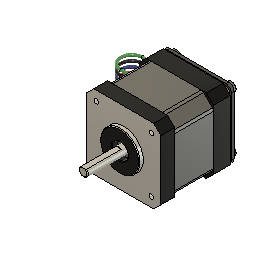
Nema 17 Closed loop v5 (Autodesk Fusion 360 design; units mm, degrees)
Autodesk Fusion 360 part; units mm, degrees
sketch "Sketch1" plane through (0, 0, 0) normal (0, 0, 1) x (1, 0, 0)
  line L0 (-20.9, 20.9) -> (20.9, 20.9)
  line L1 (20.9, 20.9) -> (20.9, -20.9)
  line L2 (20.9, -20.9) -> (-20.9, -20.9)
  line L3 (-20.9, -20.9) -> (-20.9, 20.9)
  line L4 (0, 20.9) -> (0, 0) construction
  line L5 (0, 0) -> (20.9, 0) construction
  dimension "d1" = 41.8
  dimension "d2" = 41.8
  constraint horizontal L0
  constraint vertical L1
  constraint horizontal L2
  constraint vertical L3
  constraint midpoint L0 L4.start
  constraint coincident L4.end L5.start
  constraint midpoint L1 L5.end
  constraint vertical L4
  constraint horizontal L5
  measures "d1" distance of L0.start L0.end
  measures "d2" distance of L0.end L1.end
extrude "Extrude1" add sketch "Sketch1" along normal blind 7.8 makes body 1
chamfer "Chamfer1" distance 4 angle 45 4 edges at (20.9, 20.9, 3.9) (-20.9, 20.9, 3.9) (20.9, -20.9, 3.9) (-20.9, -20.9, 3.9) on bodies 1
sketch "Sketch2" plane through (0, 0, 7.8) normal (0, 0, 1) x (1, 0, 0)
  line L0 (-20.9, -16.9) -> (-16.9, -20.9)
  line L1 (-16.9, -20.9) -> (16.9, -20.9)
  line L2 (16.9, -20.9) -> (20.9, -16.9)
  line L3 (20.9, -16.9) -> (20.9, 16.9)
  line L4 (20.9, 16.9) -> (16.9, 20.9)
  line L5 (16.9, 20.9) -> (-16.9, 20.9)
  line L6 (-16.9, 20.9) -> (-20.9, 16.9)
  line L7 (-20.9, 16.9) -> (-20.9, -16.9)
  circle A0 centre (0, 0) radius 11
  dimension "d6" = 22
  constraint coincident A0.centre origin
  measures "d6" diameter of A0
extrude "Extrude2" add sketch "Sketch2" along normal blind 2.3 contours A0 bodies 1
copy_body "Body->Comp1" bodies 1 removing the originals makes body 2 in component "Motor"
sketch "Sketch3" plane through (0, 0, 10.1) normal (0, 0, 1) x (1, 0, 0)
  circle A0 centre (0, 0) radius 4.5
  circle A1 centre (0, 0) radius 11
  dimension "d10" = 9
  constraint coincident A0.centre A1.centre
  measures "d10" diameter of A0
extrude "Extrude1'" cut sketch "Sketch3" against normal blind 3.5 contours A0 bodies 2 in component "Motor"
chamfer "Chamfer2" distance 0.4 angle 45 1 faces at (8.7924, -0.5465, 10.1) on bodies 2 in component "Motor"
sketch "Sketch4" plane through (0, 0, 6.6) normal (0, 0, 1) x (1, 0, 0)
  circle A0 centre (0, 0) radius 4.5
  circle A1 centre (0, 0) radius 2.5
  dimension "d14" = 5
  constraint coincident A0.centre A1.centre
  measures "d14" diameter of A1
extrude "Extrude3" add sketch "Sketch4" along normal blind 24 separate body contours A1 makes body 3
sketch "Sketch5" plane through (0, 0, 30.6) normal (0, 0, 1) x (1, 0, 0)
  circle A0 centre (0, 0) radius 2.5
  line L0 (-1.5, 2) -> (1.5, 2)
  line L1 (-7.396, -2.5) -> (6.5447, -2.5) construction
  dimension "d17" = 4.5
  constraint coincident A0 L0.start
  constraint coincident A0 L0.end
  constraint horizontal L0
  constraint parallel L0 L1
  constraint tangent A0 L1
  measures "d17" distance of L0 L1
extrude "Extrude4" cut sketch "Sketch5" against normal blind 20 contours A0 L0 picked at (-0.3999, 2.0645) bodies 3
chamfer "Chamfer2'" distance 0.4 angle 45 1 edges at (0, -2.5, 30.6) on bodies 3
sketch "Sketch6" plane through (0, 0, 7.8) normal (0, 0, 1) x (1, 0, 0)
  circle A0 centre (0, 0) radius 11
  line L0 (-20.9, -16.9) -> (-16.9, -20.9)
  line L1 (-16.9, -20.9) -> (16.9, -20.9)
  line L2 (16.9, -20.9) -> (20.9, -16.9)
  line L3 (20.9, -16.9) -> (20.9, 16.9)
  line L4 (20.9, 16.9) -> (16.9, 20.9)
  line L5 (16.9, 20.9) -> (-16.9, 20.9)
  line L6 (-16.9, 20.9) -> (-20.9, 16.9)
  line L7 (-20.9, 16.9) -> (-20.9, -16.9)
  circle A1 centre (-15.5, -15.5) radius 1.25
  circle A2 centre (15.5, -15.5) radius 1.25
  circle A3 centre (15.5, 15.5) radius 1.25
  circle A4 centre (-15.5, 15.5) radius 1.25
  dimension "d21" = 15.5
  dimension "d22" = 15.5
  dimension "d23" = 2.5
  dimension "d25" = 360
  measures "d21" horizontal distance of A0.centre A1.centre
  measures "d22" vertical distance of A0.centre A1.centre
  measures "d23" diameter of A1
extrude "Extrude2'" cut sketch "Sketch6" against normal blind 2.8 contours A1 | A2 | A3 | A4 bodies 2 in component "Motor"
copy_body "CutPasteBodies1" bodies 3 removing the originals makes body 4 in component "Motor"
sketch "Sketch1 (2)" plane through (0, 0, 0) normal (0, 0, -1) x (-1, 0, 0) in component "Motor"
  line L0 (16.9, -20.9) -> (20.9, -16.9)
  line L1 (20.9, -16.9) -> (20.9, 16.9)
  line L2 (20.9, 16.9) -> (16.9, 20.9)
  line L3 (16.9, 20.9) -> (-16.9, 20.9)
  line L4 (-16.9, 20.9) -> (-20.9, 16.9)
  line L5 (-20.9, 16.9) -> (-20.9, -16.9)
  line L6 (-20.9, -16.9) -> (-16.9, -20.9)
  line L7 (-16.9, -20.9) -> (16.9, -20.9)
  line L8 (-14.7787, 20.9) -> (-20.9, 14.7787)
  line L9 (-20.9, -14.7787) -> (-14.7787, -20.9)
  line L10 (14.7787, -20.9) -> (20.9, -14.7787)
  line L11 (20.9, 14.7787) -> (14.7787, 20.9)
  dimension "d28" = 1.5
  dimension "d30" = 360
  constraint coincident L3 L8.start
  constraint coincident L5 L8.end
  constraint parallel L4 L8
  measures "d28" distance of L4 L8
extrude "Extrude3'" add sketch "Sketch1 (2)" along normal blind 21.85 separate body contours L1 L3 L5 L7 L8 L9 L10 L11 makes body 5 in component "Motor"
fillet "Fillet1" radius 2 8 edges at (-14.7787, 20.9, -10.925) (-20.9, 14.7787, -10.925) (-20.9, -14.7787, -10.925) (-14.7787, -20.9, -10.925) (14.7787, 20.9, -10.925) (20.9, 14.7787, -10.925) (20.9, -14.7787, -10.925) (14.7787, -20.9, -10.925) on bodies 5 in component "Motor"
sketch "Sketch2 (2)" plane through (0, 0, -21.85) normal (0, 0, -1) x (-1, 0, 0) in component "Motor"
  arc A0 (-15.3645, -20.3142) -> (-13.9503, -20.9) centre (-13.9503, -18.9) ccw
  line L0 (-13.9503, -20.9) -> (13.9503, -20.9)
  arc A1 (13.9503, -20.9) -> (15.3645, -20.3142) centre (13.9503, -18.9) ccw
  line L1 (15.3645, -20.3142) -> (20.3142, -15.3645)
  arc A2 (20.3142, -15.3645) -> (20.9, -13.9503) centre (18.9, -13.9503) ccw
  line L2 (20.9, -13.9503) -> (20.9, 13.9503)
  arc A3 (20.9, 13.9503) -> (20.3142, 15.3645) centre (18.9, 13.9503) ccw
  line L3 (20.3142, 15.3645) -> (15.3645, 20.3142)
  arc A4 (15.3645, 20.3142) -> (13.9503, 20.9) centre (13.9503, 18.9) ccw
  line L4 (13.9503, 20.9) -> (-13.9503, 20.9)
  arc A5 (-13.9503, 20.9) -> (-15.3645, 20.3142) centre (-13.9503, 18.9) ccw
  line L5 (-15.3645, 20.3142) -> (-20.3142, 15.3645)
  arc A6 (-20.3142, 15.3645) -> (-20.9, 13.9503) centre (-18.9, 13.9503) ccw
  line L6 (-20.9, 13.9503) -> (-20.9, -13.9503)
  arc A7 (-20.9, -13.9503) -> (-20.3142, -15.3645) centre (-18.9, -13.9503) ccw
  line L7 (-20.3142, -15.3645) -> (-15.3645, -20.3142)
  line L8 (16.9, -20.9) -> (20.9, -16.9)
  line L9 (20.9, -16.9) -> (20.9, 16.9)
  line L10 (20.9, 16.9) -> (16.9, 20.9)
  line L11 (16.9, 20.9) -> (-16.9, 20.9)
  line L12 (-16.9, 20.9) -> (-20.9, 16.9)
  line L13 (-20.9, 16.9) -> (-20.9, -16.9)
  line L14 (-20.9, -16.9) -> (-16.9, -20.9)
  line L15 (-16.9, -20.9) -> (16.9, -20.9)
extrude "Extrude4'" add sketch "Sketch2 (2)" along normal blind 9.5 separate body makes body 6 in component "Motor"
sketch "Sketch3 (2)" plane through (-20.9, 0, 0) normal (-1, 0, 0) x (0, 0, 1) in component "Motor"
  line L0 (-21.85, -16.9) -> (-21.85, 16.9)
  line L1 (-21.85, 16.9) -> (-31.35, 16.9)
  line L2 (-31.35, 16.9) -> (-31.35, -16.9)
  line L3 (-31.35, -16.9) -> (-21.85, -16.9)
  line L4 (-31.35, 8.25) -> (-29.05, 8.25)
  line L5 (-29.05, 8.25) -> (-29.05, -8.25)
  line L6 (-29.05, -8.25) -> (-31.35, -8.25)
  line L7 (-31.35, -8.25) -> (-31.35, 8.25)
  line L8 (-29.05, 0) -> (0, 0) construction
  dimension "d37" = 16.5
  dimension "d38" = 2.3
  constraint horizontal L4
  constraint vertical L5
  constraint horizontal L6
  constraint vertical L7
  constraint coincident L2 L4.start
  constraint midpoint L5 L8.start
  constraint coincident L8.end origin
  constraint horizontal L8
  measures "d37" distance of L4.end L5.end
  measures "d38" distance of L4.start L4.end
extrude "Extrude5" add sketch "Sketch3 (2)" along normal blind 4 contours L2 L4 L5 L6 L7 bodies 6 in component "Motor"
sketch "Sketch4 (2)" plane through (-20.9, 0, 0) normal (-1, 0, 0) x (0, 0, 1) in component "Motor"
  line L0 (-31.35, 8.25) -> (-29.05, 8.25)
  line L1 (-29.05, 8.25) -> (-29.05, -8.25)
  line L2 (-29.05, -8.25) -> (-31.35, -8.25)
  line L3 (-31.35, -8.25) -> (-31.35, -16.9)
  line L4 (-31.35, -16.9) -> (-21.85, -16.9)
  line L5 (-21.85, -16.9) -> (-21.85, 16.9)
  line L6 (-21.85, 16.9) -> (-31.35, 16.9)
  line L7 (-31.35, 16.9) -> (-31.35, 8.25)
  line L8 (-29.05, 8.25) -> (-21.85, 8.25)
  line L9 (-21.85, 8.25) -> (-21.85, -8.25)
  line L10 (-21.85, -8.25) -> (-29.05, -8.25)
  line L11 (-29.05, -8.25) -> (-29.05, 8.25)
  constraint horizontal L8
  constraint vertical L9
  constraint horizontal L10
  constraint vertical L11
  constraint coincident L5 L9.end
  constraint coincident L0.end L1.start
  constraint collinear L2 L10
extrude "Extrude6" cut sketch "Sketch4 (2)" against normal blind 2 contours L1 L5 L8 L9 L10 L11 bodies 6 in component "Motor"
sketch "Sketch5 (2)" plane through (-18.9, 0, 0) normal (-1, 0, 0) x (0, 0, 1) in component "Motor"
  line L0 (-29.05, -8.25) -> (-21.85, -8.25)
  line L1 (-21.85, -8.25) -> (-21.85, 8.25)
  line L2 (-21.85, 8.25) -> (-29.05, 8.25)
  line L3 (-29.05, 8.25) -> (-29.05, -8.25)
  line L4 (-28.55, 7.75) -> (-22.35, 7.75)
  line L5 (-22.35, 7.75) -> (-22.35, -7.75)
  line L6 (-22.35, -7.75) -> (-28.55, -7.75)
  line L7 (-28.55, -7.75) -> (-28.55, 7.75)
  dimension "d43" = 0.5
  dimension "d44" = 0.5
  dimension "d45" = 0.5
  dimension "d46" = 0.5
  constraint horizontal L4
  constraint vertical L5
  constraint horizontal L6
  constraint vertical L7
  measures "d43" distance of L3 L7
  measures "d44" distance of L1 L5
  measures "d45" distance of L2 L4
  measures "d46" distance of L0 L6
extrude "Extrude7" add sketch "Sketch5 (2)" along normal blind 5 separate body contours L4 L5 L6 L7 makes body 7 in component "Motor"
sketch "Sketch6 (2)" plane through (0, 0, -31.35) normal (0, 0, -1) x (-1, 0, 0) in component "Motor"
  line L0 (-16.9, -20.9) -> (16.9, -20.9)
  line L1 (16.9, -20.9) -> (20.9, -16.9)
  line L2 (20.9, -16.9) -> (20.9, -8.25)
  line L3 (20.9, -8.25) -> (24.9, -8.25)
  line L4 (24.9, -8.25) -> (24.9, 8.25)
  line L5 (24.9, 8.25) -> (20.9, 8.25)
  line L6 (20.9, 8.25) -> (20.9, 16.9)
  line L7 (20.9, 16.9) -> (16.9, 20.9)
  line L8 (16.9, 20.9) -> (-16.9, 20.9)
  line L9 (-16.9, 20.9) -> (-20.9, 16.9)
  line L10 (-20.9, 16.9) -> (-20.9, -16.9)
  line L11 (-20.9, -16.9) -> (-16.9, -20.9)
  circle A0 centre (15.5, 15.5) radius 3.25
  circle A1 centre (15.5, 15.5) radius 1.25
  circle A2 centre (-15.5, 15.5) radius 3.25
  circle A3 centre (-15.5, -15.5) radius 3.25
  circle A4 centre (15.5, -15.5) radius 3.25
  dimension "d49" = 6.5
  dimension "d51" = 360
  constraint concentric A0 A1
  measures "d49" diameter of A0
extrude "Extrude8" add sketch "Sketch6 (2)" along normal blind 1.9 separate body contours A0 | A1 | A2 | A3 | A4 makes body 8 at (12.254, -15.662, -32.6167) makes body 9 at (12.254, 15.338, -32.6167) makes body 10 at (-18.746, -15.662, -32.6167) makes body 11 at (-18.746, 15.338, -32.6167) in component "Motor"
sketch "Sketch7" plane through (0, 0, -33.25) normal (0, 0, -1) x (-1, 0, 0) in component "Motor"
  circle A0 centre (15.5, 15.5) radius 3.25
  line L0 (-16.5, 19.5) -> (16.5, 19.5)
  line L1 (19.5, 16.5) -> (19.5, -16.5)
  line L2 (16.5, -19.5) -> (-16.5, -19.5)
  line L3 (-19.5, -16.5) -> (-19.5, 16.5)
  line L4 (16.9, 20.9) -> (-16.9, 20.9)
  line L5 (-16.9, -20.9) -> (16.9, -20.9)
  line L6 (-20.9, 16.9) -> (-20.9, -16.9)
  arc A1 (19.5, 16.5) -> (16.5, 19.5) centre (16.5, 16.5) ccw
  arc A2 (16.5, -19.5) -> (19.5, -16.5) centre (16.5, -16.5) ccw
  arc A3 (-19.5, -16.5) -> (-16.5, -19.5) centre (-16.5, -16.5) ccw
  arc A4 (-16.5, 19.5) -> (-19.5, 16.5) centre (-16.5, 16.5) ccw
  point P0 (-19.5, 19.5)
  point P1 (19.5, 19.5)
  point P2 (19.5, -19.5)
  dimension "d54" = 39
  dimension "d55" = 39
  dimension "d56" = 1.4
  dimension "d57" = 1.4
  dimension "d58" = 1.4
  dimension "d59" = 3
  constraint horizontal L0
  constraint vertical L1
  constraint horizontal L2
  constraint vertical L3
  constraint coincident P1 L0
  constraint coincident P1 L1
  constraint tangent L0 A1
  constraint tangent L1 A1
  constraint coincident P2 L1
  constraint coincident P2 L2
  constraint tangent L1 A2
  constraint tangent L2 A2
  constraint equal A1 A2
  constraint tangent L2 A3
  constraint tangent L3 A3
  constraint equal A1 A3
  constraint coincident P0 L0
  constraint coincident P0 L3
  constraint tangent L0 A4
  constraint tangent L3 A4
  constraint equal A1 A4
  measures "d54" distance of P0 P1
  measures "d55" distance of P1 P2
  measures "d56" distance of L0 L4
  measures "d57" distance of L2 L5
  measures "d58" distance of L3 L6
  measures "d59" radius of A1
extrude "Extrude9" add sketch "Sketch7" along normal blind 1.6 separate body contours A0 | L0 L1 L2 L3 A1 A2 A3 A4 makes body 12 in component "Motor"
sketch "Sketch8" plane through (0, 0, -34.85) normal (0, 0, -1) x (-1, 0, 0) in component "Motor"
  arc A0 (19.5, 16.5) -> (16.5, 19.5) centre (16.5, 16.5) ccw
  line L0 (16.5, 19.5) -> (-16.5, 19.5)
  arc A1 (-16.5, 19.5) -> (-19.5, 16.5) centre (-16.5, 16.5) ccw
  line L1 (-19.5, 16.5) -> (-19.5, -16.5)
  arc A2 (-19.5, -16.5) -> (-16.5, -19.5) centre (-16.5, -16.5) ccw
  line L2 (-16.5, -19.5) -> (16.5, -19.5)
  arc A3 (16.5, -19.5) -> (19.5, -16.5) centre (16.5, -16.5) ccw
  line L3 (19.5, -16.5) -> (19.5, 16.5)
  line L4 (18.4811, 6.25) -> (23.9, 6.25)
  line L5 (23.9, 6.25) -> (23.9, -6.25)
  line L6 (23.9, -6.25) -> (18.4811, -6.25)
  line L7 (18.4811, -6.25) -> (18.4811, 6.25)
  line L8 (23.9, 7.75) -> (23.9, -7.75)
  line L9 (0, 0) -> (18.4811, 0) construction
  dimension "d62" = 12.5
  dimension "d63" = 5.4189
  constraint horizontal L4
  constraint vertical L5
  constraint horizontal L6
  constraint vertical L7
  constraint collinear L5 L8
  constraint coincident L9.start origin
  constraint midpoint L7 L9.end
  constraint horizontal L9
  measures "d62" distance of L4.start L6.end
  measures "d63" distance of L4.start L4.end
extrude "Extrude10" add sketch "Sketch8" along normal blind 5.6 separate body contours L3 L4 L5 L6 L8 | L3 L4 L6 L7 makes body 13 in component "Motor"
ref_plane "WorkPlane1" through (-21.1906, -4.25, -37.65) normal (0, -1, 0) x (-1, 0, 0) in component "Motor"
sketch "Sketch9" plane through (-21.1906, -4.25, -37.65) normal (0, -1, 0) x (1, 0, 0) in component "Motor"
  line L0 (-2.7094, 0) -> (-13.6094, 0)
  line L1 (-2.7094, 12.2) -> (-13.6094, 12.2)
  line L2 (2.2906, 15.3) -> (-2.7094, 15.3)
  line L3 (2.7094, -2.8) -> (-2.7094, -2.8)
  line L4 (-2.7094, 9.1) -> (-2.7094, 15.3)
  line L5 (-2.7094, 2.8) -> (-2.7094, -2.8)
  arc A0 (-13.6094, 12.2) -> (-13.6094, 0) centre (-13.6094, 6.1) ccw
  line L6 (0.2906, 15.8) -> (0.2906, 6.3)
  point P0 (-19.7094, 6.1)
  dimension "d67" = 3.1
  dimension "d68" = 2.8
  dimension "d69" = 20
  constraint horizontal L0
  constraint parallel L0 L1
  constraint coincident L1.start L4
  constraint coincident L0.start L5
  constraint vertical L0.end L1.end
  constraint tangent L1 A0
  constraint midpoint A0 P0
  measures "d67" distance of L1 L2
  measures "d68" distance of L0 L3
  measures "d69" distance of P0 L6
sketch "Sketch10" plane through (-23.9, 0, 0) normal (-1, 0, 0) x (0, 0, 1) in component "Motor"
  line L0 (-34.85, -6.25) -> (-34.85, 6.25)
  line L1 (-34.85, 6.25) -> (-40.45, 6.25)
  line L2 (-40.45, 6.25) -> (-40.45, -6.25)
  line L3 (-40.45, -6.25) -> (-34.85, -6.25)
  circle A0 centre (-37.65, -4.25) radius 0.75
  point P0 (-37.65, -4.25)
  dimension "d70" = 1.5
  constraint coincident P0 A0.centre
  measures "d70" diameter of A0
sweep "Sweep1" add profiles "Sketch10" path "Sketch9" along L0 A0 L1 section 1 contours A0 separate body makes body 14 in component "Motor"
pattern_linear "R-Pattern1" count 4 spacing 2.9113 along (0, 1, 0) of bodies 14 makes body 15 at (-38.3482, -1.0822, -37.3564) makes body 16 at (-38.3482, 1.8292, -37.3564) makes body 17 at (-38.3482, 4.7405, -37.3564) in component "Motor"
sketch "Sketch11" plane through (0, 0, -34.85) normal (0, 0, -1) x (-1, 0, 0) in component "Motor"
  arc A0 (19.5, 16.5) -> (16.5, 19.5) centre (16.5, 16.5) ccw
  line L0 (16.5, 19.5) -> (-16.5, 19.5)
  arc A1 (-16.5, 19.5) -> (-19.5, 16.5) centre (-16.5, 16.5) ccw
  line L1 (-19.5, 16.5) -> (-19.5, -16.5)
  arc A2 (-19.5, -16.5) -> (-16.5, -19.5) centre (-16.5, -16.5) ccw
  line L2 (-16.5, -19.5) -> (16.5, -19.5)
  arc A3 (16.5, -19.5) -> (19.5, -16.5) centre (16.5, -16.5) ccw
  line L3 (19.5, -16.5) -> (19.5, 16.5)
  circle A4 centre (-15.5, 15.5) radius 2.725
  circle A5 centre (-15.5, -15.5) radius 2.725
  circle A6 centre (15.5, -15.5) radius 2.725
  circle A7 centre (15.5, 15.5) radius 2.725
  dimension "d81" = 5.45
  dimension "d82" = 4
  dimension "d83" = 4
  dimension "d85" = 360
  measures "d81" diameter of A4
  measures "d82" distance of L0 A4.centre
  measures "d83" distance of L1 A4.centre
extrude "Extrude11" add sketch "Sketch11" along normal blind 2.7 separate body contours A4 | A5 | A6 | A7 makes body 18 at (12.7784, 15.3642, -36.65) makes body 19 at (12.7784, -15.6358, -36.65) makes body 20 at (-18.2216, 15.3642, -36.65) makes body 21 at (-18.2216, -15.6358, -36.65) in component "Motor"
chamfer "Chamfer3" distance 0.3 angle 45 4 faces at (12.7784, -15.6358, -36.65) (12.7784, 15.3642, -36.65) (-18.2216, 15.3642, -36.65) (-18.2216, -15.6358, -36.65) on bodies 18 19 20 21 in component "Motor"
sketch "Sketch12" plane through (0, 0, -37.55) normal (0, 0, -1) x (-1, 0, 0) in component "Motor"
  circle A0 centre (-15.5, 15.5) radius 2.425
  line L0 (-14.25, 14.7783) -> (-14.25, 16.2217)
  line L1 (-14.25, 16.2217) -> (-15.5, 16.9434)
  line L2 (-15.5, 16.9434) -> (-16.75, 16.2217)
  line L3 (-16.75, 16.2217) -> (-16.75, 14.7783)
  line L4 (-16.75, 14.7783) -> (-15.5, 14.0566)
  line L5 (-15.5, 14.0566) -> (-14.25, 14.7783)
  line L6 (-16.9434, -15.5) -> (-16.2217, -16.75)
  line L7 (-16.2217, -14.25) -> (-16.9434, -15.5)
  line L8 (-14.7783, -14.25) -> (-16.2217, -14.25)
  line L9 (-14.0566, -15.5) -> (-14.7783, -14.25)
  line L10 (-14.7783, -16.75) -> (-14.0566, -15.5)
  line L11 (-16.2217, -16.75) -> (-14.7783, -16.75)
  line L12 (15.5, -16.9434) -> (16.75, -16.2217)
  line L13 (14.25, -16.2217) -> (15.5, -16.9434)
  line L14 (14.25, -14.7783) -> (14.25, -16.2217)
  line L15 (15.5, -14.0566) -> (14.25, -14.7783)
  line L16 (16.75, -14.7783) -> (15.5, -14.0566)
  line L17 (16.75, -16.2217) -> (16.75, -14.7783)
  line L18 (16.9434, 15.5) -> (16.2217, 16.75)
  line L19 (16.2217, 14.25) -> (16.9434, 15.5)
  line L20 (14.7783, 14.25) -> (16.2217, 14.25)
  line L21 (14.0566, 15.5) -> (14.7783, 14.25)
  line L22 (14.7783, 16.75) -> (14.0566, 15.5)
  line L23 (16.2217, 16.75) -> (14.7783, 16.75)
  point P0 (-15.5, 15.5)
  point P1 (-15.5, -15.5)
  point P2 (-15.5, -15.5)
  point P3 (15.5, -15.5)
  point P4 (15.5, -15.5)
  point P5 (15.5, 15.5)
  point P6 (15.5, 15.5)
  dimension "d89" = 2.5
  dimension "d91" = 360
  constraint coincident P0 A0.centre
  constraint vertical L0
  measures "d89" distance of L0 L3
extrude "Extrude12" cut sketch "Sketch12" against normal blind 2 contours L0 L1 L2 L3 L4 L5 | L6 L7 L8 L9 L10 L11 | L12 L13 L14 L15 L16 L17 | L18 L19 L20 L21 L22 L23 bodies 18 19 20 21 in component "Motor"
sketch "Sketch13" plane through (0, 0, -34.85) normal (0, 0, -1) x (-1, 0, 0) in component "Motor"
  arc A0 (19.5, 16.5) -> (16.5, 19.5) centre (16.5, 16.5) ccw
  line L0 (16.5, 19.5) -> (-16.5, 19.5)
  arc A1 (-16.5, 19.5) -> (-19.5, 16.5) centre (-16.5, 16.5) ccw
  line L1 (-19.5, 16.5) -> (-19.5, -16.5)
  arc A2 (-19.5, -16.5) -> (-16.5, -19.5) centre (-16.5, -16.5) ccw
  line L2 (-16.5, -19.5) -> (16.5, -19.5)
  arc A3 (16.5, -19.5) -> (19.5, -16.5) centre (16.5, -16.5) ccw
  line L3 (19.5, -16.5) -> (19.5, 16.5)
  line L4 (-8.75, -16.7) -> (8.75, -16.7)
  line L5 (8.75, -16.7) -> (8.75, -23.7)
  line L6 (8.75, -23.7) -> (-8.75, -23.7)
  line L7 (-8.75, -23.7) -> (-8.75, -16.7)
  line L8 (0, -16.7) -> (0, 0) construction
  line L9 (-16.9, -20.9) -> (16.9, -20.9)
  dimension "d94" = 17.5
  dimension "d95" = 7
  dimension "d96" = 2.8
  constraint horizontal L4
  constraint vertical L5
  constraint horizontal L6
  constraint vertical L7
  constraint midpoint L4 L8.start
  constraint coincident L8.end origin
  constraint vertical L8
  measures "d94" distance of L4.start L4.end
  measures "d95" distance of L4.end L5.end
  measures "d96" distance of L6 L9
extrude "Extrude13" add sketch "Sketch13" along normal blind 5.7 separate body contours L2 L5 L7 L9 | L2 L4 L5 L7 | L5 L6 L7 L9 makes body 22 in component "Motor"
sketch "Sketch14" plane through (0, -23.7, 0) normal (0, -1, 0) x (1, 0, 0) in component "Motor"
  line L0 (8.75, -34.85) -> (-8.75, -34.85)
  line L1 (-8.75, -34.85) -> (-8.75, -40.55)
  line L2 (-8.75, -40.55) -> (8.75, -40.55)
  line L3 (8.75, -40.55) -> (8.75, -34.85)
  line L4 (-8.05, -35.55) -> (8.05, -35.55)
  line L5 (8.05, -35.55) -> (8.05, -39.85)
  line L6 (-8.05, -39.85) -> (-8.05, -35.55)
  line L7 (-5, -39.85) -> (-5, -40.55)
  line L8 (-5, -40.55) -> (-6.5, -40.55)
  line L9 (-6.5, -40.55) -> (-6.5, -39.85)
  line L10 (6.5, -39.85) -> (6.5, -40.55)
  line L11 (6.5, -40.55) -> (5, -40.55)
  line L12 (5, -40.55) -> (5, -39.85)
  line L13 (-6.5, -39.85) -> (-8.05, -39.85)
  line L14 (8.05, -39.85) -> (6.5, -39.85)
  line L15 (5, -39.85) -> (-5, -39.85)
  dimension "d99" = 0.7
  dimension "d100" = 0.7
  dimension "d101" = 0.7
  dimension "d102" = 0.7
  dimension "d103" = 1.5
  dimension "d104" = 1.5
  dimension "d105" = 10
  constraint horizontal L4
  constraint vertical L5
  constraint horizontal L14
  constraint vertical L6
  constraint vertical L7
  constraint horizontal L8
  constraint vertical L9
  constraint coincident L2 L7.end
  constraint coincident L9.end L14
  constraint vertical L10
  constraint horizontal L11
  constraint vertical L12
  constraint coincident L2 L10.end
  constraint coincident L12.end L14
  constraint collinear L13 L14
  constraint collinear L14 L15
  constraint equal L13 L14
  measures "d99" distance of L1 L6
  measures "d100" distance of L3 L5
  measures "d101" distance of L2 L14
  measures "d102" distance of L0 L4
  measures "d103" distance of L10.end L11.end
  measures "d104" distance of L7.end L8.end
  measures "d105" distance of L7.start L12.end
extrude "Extrude14" cut sketch "Sketch14" against normal blind 5.5 contours L2 L4 L5 L6 L7 L8 L9 L10 L11 L12 L13 L14 L15 bodies 22 in component "Motor"
sketch "Sketch15" plane through (0, 0, -34.85) normal (0, 0, -1) x (-1, 0, 0) in component "Motor"
  arc A0 (19.5, 16.5) -> (16.5, 19.5) centre (16.5, 16.5) ccw
  line L0 (16.5, 19.5) -> (-16.5, 19.5)
  arc A1 (-16.5, 19.5) -> (-19.5, 16.5) centre (-16.5, 16.5) ccw
  line L1 (-19.5, 16.5) -> (-19.5, -16.5)
  arc A2 (-19.5, -16.5) -> (-16.5, -19.5) centre (-16.5, -16.5) ccw
  line L2 (-16.5, -19.5) -> (16.5, -19.5)
  arc A3 (16.5, -19.5) -> (19.5, -16.5) centre (16.5, -16.5) ccw
  line L3 (19.5, -16.5) -> (19.5, 16.5)
  line L4 (-2.5, 6) -> (5.5, 6)
  line L5 (5.5, 6) -> (5.5, -6)
  line L6 (5.5, -6) -> (-2.5, -6)
  line L7 (-2.5, -6) -> (-2.5, 6)
  dimension "d108" = 12
  dimension "d109" = 8
  dimension "d110" = 6
  dimension "d111" = 14
  constraint horizontal L4
  constraint vertical L5
  constraint horizontal L6
  constraint vertical L7
  measures "d108" distance of L4.start L6.end
  measures "d109" distance of L5.end L6.end
  measures "d110" distance of origin L6
  measures "d111" distance of L3 L5
extrude "Extrude15" add sketch "Sketch15" along normal blind 1.5 contours L4 L5 L6 L7 bodies 12 in component "Motor"
component "Motor" placed x (1, 0, 0) y (0, 1, 0) z (0, 0, 1) at (0, 0, 0)
equation "d25 = 360.0 °"
equation "d30 = 360.0 °"
equation "d51 = 360.0 °"
equation "d85 = 360.0 °"
equation "d91 = 360.0 °"
named bodies: "Front cover", "Shaft", "Middle body", "Back cover", "Connector", "Driver board"
